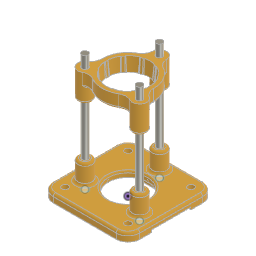
Drill_Guide_v7 (Autodesk Fusion 360 design; units mm, degrees)
Autodesk Fusion 360 part; units mm, degrees
sketch "Sketch1" plane through (0, 0, 0) normal (0, 0, 1) x (1, 0, 0) in component "Mount"
  circle A0 centre (0, 0) radius 32.75
  dimension "d45" = 65.5
  constraint coincident A0.centre origin
  measures "d45" diameter of A0
extrude "Extrude1" add sketch "Sketch1" along normal blind 17 makes body 1 in component "Mount"
sketch "Sketch3" plane through (0, 0, 0) normal (0, 0, -1) x (1, 0, 0) in component "Mount"
  circle A0 centre (0, 0) radius 32.75
  circle A1 centre (0, 0) radius 27.75
  line L0 (0, 0) -> (-27.75, 0) construction
  line L1 (-28.25, -2.5) -> (-28.25, -2.5)
  line L2 (-27.25, -1.5) -> (-27.25, 1.5)
  line L3 (-28.25, 2.5) -> (-28.25, 2.5)
  line L4 (-28.25, 2.5) -> (-28.25, -2.5)
  line L5 (-28.25, -2.5) -> (-27.25, 2.5) construction
  line L6 (-27.25, -2.5) -> (-28.25, 2.5) construction
  arc A2 (-27.25, 1.5) -> (-28.25, 2.5) centre (-28.25, 1.5) ccw
  arc A3 (-28.25, -2.5) -> (-27.25, -1.5) centre (-28.25, -1.5) ccw
  line L7 (-21.164, -17.2307) -> (-22.9274, -14.8036)
  arc A4 (-21.3853, -18.6275) -> (-21.164, -17.2307) centre (-21.9731, -17.8185) ccw
  arc A5 (-22.9274, -14.8036) -> (-24.3242, -14.5824) centre (-23.7364, -15.3914) ccw
  line L8 (-24.3242, -14.5824) -> (-21.3853, -18.6275)
  line L9 (-6.9941, -26.3798) -> (-9.8473, -25.4528)
  arc A6 (-6.3521, -27.6399) -> (-6.9941, -26.3798) centre (-7.3031, -27.3309) ccw
  arc A7 (-9.8473, -25.4528) -> (-11.1074, -26.0948) centre (-10.1563, -26.4038) ccw
  line L10 (-11.1074, -26.0948) -> (-6.3521, -27.6399)
  line L11 (9.8473, -25.4528) -> (6.9941, -26.3798)
  arc A8 (11.1074, -26.0948) -> (9.8473, -25.4528) centre (10.1563, -26.4038) ccw
  arc A9 (6.9941, -26.3798) -> (6.3521, -27.6399) centre (7.3031, -27.3309) ccw
  line L12 (6.3521, -27.6399) -> (11.1074, -26.0948)
  line L13 (22.9274, -14.8036) -> (21.164, -17.2307)
  arc A10 (24.3242, -14.5824) -> (22.9274, -14.8036) centre (23.7364, -15.3914) ccw
  arc A11 (21.164, -17.2307) -> (21.3853, -18.6275) centre (21.9731, -17.8185) ccw
  line L14 (21.3853, -18.6275) -> (24.3242, -14.5824)
  line L15 (27.25, 1.5) -> (27.25, -1.5)
  arc A12 (28.25, 2.5) -> (27.25, 1.5) centre (28.25, 1.5) ccw
  arc A13 (27.25, -1.5) -> (28.25, -2.5) centre (28.25, -1.5) ccw
  line L16 (28.25, -2.5) -> (28.25, 2.5)
  line L17 (21.164, 17.2307) -> (22.9274, 14.8036)
  arc A14 (21.3853, 18.6275) -> (21.164, 17.2307) centre (21.9731, 17.8185) ccw
  arc A15 (22.9274, 14.8036) -> (24.3242, 14.5824) centre (23.7364, 15.3914) ccw
  line L18 (24.3242, 14.5824) -> (21.3853, 18.6275)
  line L19 (6.9941, 26.3798) -> (9.8473, 25.4528)
  arc A16 (6.3521, 27.6399) -> (6.9941, 26.3798) centre (7.3031, 27.3309) ccw
  arc A17 (9.8473, 25.4528) -> (11.1074, 26.0948) centre (10.1563, 26.4038) ccw
  line L20 (11.1074, 26.0948) -> (6.3521, 27.6399)
  line L21 (-9.8473, 25.4528) -> (-6.9941, 26.3798)
  arc A18 (-11.1074, 26.0948) -> (-9.8473, 25.4528) centre (-10.1563, 26.4038) ccw
  arc A19 (-6.9941, 26.3798) -> (-6.3521, 27.6399) centre (-7.3031, 27.3309) ccw
  line L22 (-6.3521, 27.6399) -> (-11.1074, 26.0948)
  line L23 (-22.9274, 14.8036) -> (-21.164, 17.2307)
  arc A20 (-24.3242, 14.5824) -> (-22.9274, 14.8036) centre (-23.7364, 15.3914) ccw
  arc A21 (-21.164, 17.2307) -> (-21.3853, 18.6275) centre (-21.9731, 17.8185) ccw
  line L24 (-21.3853, 18.6275) -> (-24.3242, 14.5824)
  point P0 (-27.75, 0)
  dimension "d60" = 55.5
  dimension "d61" = 1
  dimension "d62" = 5
  dimension "d63" = 1
  dimension "d64" = 1
  dimension "d66" = 360
  constraint coincident A0.centre A1.centre
  constraint coincident A1 P0
  constraint horizontal L0
  constraint parallel L2 L4
  constraint coincident L5 P0
  constraint coincident L6 P0
  constraint coincident P0 L0.end
  constraint coincident L5.end L3
  constraint coincident L5.end L2
  constraint tangent L2 A2
  constraint coincident L6.start L1
  constraint coincident L6.start L2
  constraint tangent L2 A3
  measures "d60" diameter of A1
  measures "d61" distance of L5.end L3.start
  measures "d62" distance of L6.start L5.end
  measures "d63" radius of A2
  measures "d64" radius of A3
extrude "Extrude2" cut sketch "Sketch3" against normal up to surface (17 mm away) draft -5 contours A1 L2 A2 A3 L7 A4 A5 L9 A6 A7 L11 A8 A9 L13 A10 A11 L15 A12 A13 L17 A14 A15 L19 A16 A17 L21 A18 A19 L23 A20 A21 bodies 1 in component "Mount"
sketch "Sketch1 (2)" plane through (0, 0, 0) normal (0, 0, 1) x (1, 0, 0) in component "Base"
  circle A0 centre (-40, -40) radius 4
  line L0 (-55, 55) -> (55, -55) construction
  line L1 (55, 55) -> (-55, -55) construction
  arc A1 (-40, 55) -> (-55, 40) centre (-40, 40) ccw
  arc A2 (-55, -40) -> (-40, -55) centre (-40, -40) ccw
  line L2 (-55, -40) -> (-55, 40)
  circle A3 centre (-40, 40) radius 4
  line L3 (-40, 55) -> (40, 55)
  arc A4 (55, 40) -> (40, 55) centre (40, 40) ccw
  line L4 (55, 40) -> (55, -40)
  line L5 (40, -55) -> (-40, -55)
  circle A5 centre (40, -40) radius 4
  arc A6 (40, -55) -> (55, -40) centre (40, -40) ccw
  circle A7 centre (40, 40) radius 4
  circle A8 centre (0, 0) radius 25
  dimension "d69" = 110
  dimension "d70" = 110
  dimension "d71" = 15
  dimension "d72" = 15
  dimension "d73" = 15
  dimension "d74" = 15
  dimension "d75" = 8
  dimension "d76" = 8
  dimension "d77" = 8
  dimension "d78" = 8
  dimension "d79" = 50
  constraint horizontal L3
  constraint perpendicular L3 L4
  constraint parallel L3 L5
  constraint parallel L2 L4
  constraint coincident A8.centre L0
  constraint coincident A8.centre L1
  constraint coincident A8.centre origin
  constraint coincident L1.end L2
  constraint coincident L1.end L5
  constraint tangent A2 L2
  constraint tangent A2 L5
  constraint coincident L0.start L2
  constraint coincident L0.start L3
  constraint tangent A1 L2
  constraint tangent A1 L3
  constraint coincident L1.start L3
  constraint coincident L1.start L4
  constraint tangent L3 A4
  constraint tangent A4 L4
  constraint coincident L0.end L4
  constraint coincident L0.end L5
  constraint tangent L4 A6
  constraint tangent L5 A6
  constraint concentric A0 A2
  constraint concentric A5 A6
  constraint concentric A4 A7
  constraint concentric A1 A3
  measures "d69" distance of L0.end L1.end
  measures "d70" distance of L0.end L1.start
  measures "d71" radius of A2
  measures "d72" radius of A1
  measures "d73" radius of A4
  measures "d74" radius of A6
  measures "d75" diameter of A0
  measures "d76" diameter of A5
  measures "d77" diameter of A7
  measures "d78" diameter of A3
  measures "d79" diameter of A8
extrude "Extrude1'" add sketch "Sketch1 (2)" along normal blind 10 separate body makes body 2 in component "Base"
sketch "Sketch2" plane through (55, 0, 0) normal (1, 0, 0) x (0, 1, 0) in component "Base"
  line L0 (-40, 0) -> (40, 0)
  line L1 (40, 0) -> (40, 10)
  line L2 (40, 10) -> (-40, 10)
  line L3 (-40, 10) -> (-40, 0)
  line L4 (25, 0) -> (-25, 0)
  line L5 (25, 3) -> (25, 0)
  line L6 (-40, 0) -> (40, 0)
  line L7 (40, 0) -> (40, 10)
  line L8 (40, 10) -> (-40, 10)
  line L9 (-40, 10) -> (-40, 0)
  line L10 (-25, 0) -> (-25, 3)
  line L11 (-25, 3) -> (25, 3)
  dimension "d82" = 50
  dimension "d83" = 3
  constraint horizontal L11
  constraint vertical L5
  constraint horizontal L4
  constraint vertical L10
  constraint midpoint origin L4
  measures "d82" distance of L10.end L5.start
  measures "d83" distance of L10.end L4.end
extrude "Extrude2'" cut sketch "Sketch2" against normal up to surface (110 mm away) contours L0 L4 L5 L6 L10 L11 bodies 2 in component "Base"
sketch "Sketch3 (2)" plane through (0, 0, 10) normal (0, 0, 1) x (-1, 0, 0) in component "Base"
  circle A0 centre (-40, -40) radius 4
  circle A1 centre (0, 0) radius 25
  circle A2 centre (40, 40) radius 4
  circle A3 centre (40, -40) radius 4
  circle A4 centre (-40, 40) radius 4
  arc A5 (55, 40) -> (40, 55) centre (40, 40) ccw
  line L0 (40, 55) -> (-40, 55)
  arc A6 (-40, 55) -> (-55, 40) centre (-40, 40) ccw
  line L1 (-55, 40) -> (-55, -40)
  arc A7 (-55, -40) -> (-40, -55) centre (-40, -40) ccw
  line L2 (-40, -55) -> (40, -55)
  arc A8 (40, -55) -> (55, -40) centre (40, -40) ccw
  line L3 (55, -40) -> (55, 40)
  circle A9 centre (0, 0) radius 25
  circle A10 centre (40, 40) radius 4
  circle A11 centre (-40, 40) radius 4
  circle A12 centre (-40, -40) radius 4
  arc A13 (40, -55) -> (55, -40) centre (40, -40) ccw
  circle A14 centre (0, -40) radius 9
  circle A15 centre (-34.641, 20) radius 9
  circle A16 centre (34.641, 20) radius 9
  line L4 (-40, -55) -> (40, -55)
  circle A17 centre (40, -40) radius 4
  line L5 (40, 55) -> (-40, 55)
  line L6 (55, -40) -> (55, 40)
  arc A18 (55, 40) -> (40, 55) centre (40, 40) ccw
  arc A19 (-40, 55) -> (-55, 40) centre (-40, 40) ccw
  line L7 (-55, 40) -> (-55, -40)
  arc A20 (-55, -40) -> (-40, -55) centre (-40, -40) ccw
  dimension "d87" = 360
  dimension "d88" = 40
  dimension "d89" = 55
  measures "d88" distance of A14.centre A1.centre
  measures "d89" distance of A14.centre L6
extrude "Extrude3" add sketch "Sketch3 (2)" along normal blind 25 contours A14 | A15 | A16 bodies 2 in component "Base"
sketch "Sketch4" plane through (0, 0, 35) normal (0, 0, 1) x (-1, 0, 0) in component "Base"
  circle A0 centre (0, -40) radius 9
  circle A1 centre (34.641, 20) radius 4
  circle A2 centre (-34.641, 20) radius 4
  circle A3 centre (0, -40) radius 4
  circle A4 centre (0, -40) radius 9
  dimension "d93" = 360
  dimension "d94" = 8
  constraint concentric A3 A4
  measures "d94" diameter of A3
extrude "Extrude4" cut sketch "Sketch4" against normal up to surface (35 mm away) contours A1 | A2 | A3 bodies 2 in component "Base"
ref_plane "WorkPlane1" through (0, 0, 3) normal (0, 0, 1) x (1, 0, 0) in component "Base"
sketch "Sketch5" plane through (0, 0, 3) normal (0, 0, 1) x (1, 0, 0) in component "Base"
  circle A0 centre (25, 0) radius 0.5
  circle A1 centre (0, -25) radius 0.5
  circle A2 centre (0, 25) radius 0.5
  circle A3 centre (-25, 0) radius 0.5
  dimension "d99" = 360
  dimension "d100" = 1
  measures "d100" diameter of A2
extrude "Extrude5" add sketch "Sketch5" along normal blind 3 bodies 2 in component "Base"
fillet "Fillet1" radius 3 11 edges at (55, 0, 10) (50.6066, 50.6066, 10) (0, 55, 10) (-50.6066, 50.6066, 10) (-55, 0, 10) (-50.6066, -50.6066, 10) (0, -55, 10) (50.6066, -50.6066, 10) (43.032, -16.7455, 35) (8.3909, 43.2545, 35) (-26.2501, -16.7455, 35) on bodies 2 in component "Base"
fillet "Fillet3" radius 2 1 edges at (-23.3082, 9.0404, 10) on bodies 2 in component "Base"
fillet "Fillet4" radius 3 3 edges at (-26.2501, -23.2545, 10) (8.3909, 36.7455, 10) (43.032, -23.2545, 10) on bodies 2 in component "Base"
sketch "Sketch4 (2)" plane through (0, 0, 0) normal (0, 0, -1) x (1, 0, 0) in component "Mount"
  arc A0 (23.7265, -14.3915) -> (27.6543, -2.3032) centre (0, 0) ccw
  arc A1 (23.7265, -14.3915) -> (22.9274, -14.8036) centre (23.7364, -15.3914) ccw
  line L0 (22.9274, -14.8036) -> (21.164, -17.2307)
  arc A2 (21.164, -17.2307) -> (21.019, -18.1181) centre (21.9731, -17.8185) ccw
  arc A3 (10.7361, -25.589) -> (21.019, -18.1181) centre (0, 0) ccw
  arc A4 (10.7361, -25.589) -> (9.8473, -25.4528) centre (10.1563, -26.4038) ccw
  line L1 (9.8473, -25.4528) -> (6.9941, -26.3798)
  arc A5 (6.9941, -26.3798) -> (6.3552, -27.0125) centre (7.3031, -27.3309) ccw
  arc A6 (-6.3552, -27.0125) -> (6.3552, -27.0125) centre (0, 0) ccw
  arc A7 (-6.3552, -27.0125) -> (-6.9941, -26.3798) centre (-7.3031, -27.3309) ccw
  line L2 (-6.9941, -26.3798) -> (-9.8473, -25.4528)
  arc A8 (-9.8473, -25.4528) -> (-10.7361, -25.589) centre (-10.1563, -26.4038) ccw
  arc A9 (-21.019, -18.1181) -> (-10.7361, -25.589) centre (0, 0) ccw
  arc A10 (-21.019, -18.1181) -> (-21.164, -17.2307) centre (-21.9731, -17.8185) ccw
  line L3 (-21.164, -17.2307) -> (-22.9274, -14.8036)
  arc A11 (-22.9274, -14.8036) -> (-23.7265, -14.3915) centre (-23.7364, -15.3914) ccw
  arc A12 (-27.6543, -2.3032) -> (-23.7265, -14.3915) centre (0, 0) ccw
  arc A13 (-27.6543, -2.3032) -> (-27.25, -1.5) centre (-28.25, -1.5) ccw
  line L4 (-27.25, -1.5) -> (-27.25, 1.5)
  arc A14 (-27.25, 1.5) -> (-27.6543, 2.3032) centre (-28.25, 1.5) ccw
  arc A15 (-23.7265, 14.3915) -> (-27.6543, 2.3032) centre (0, 0) ccw
  arc A16 (-23.7265, 14.3915) -> (-22.9274, 14.8036) centre (-23.7364, 15.3914) ccw
  line L5 (-22.9274, 14.8036) -> (-21.164, 17.2307)
  arc A17 (-21.164, 17.2307) -> (-21.019, 18.1181) centre (-21.9731, 17.8185) ccw
  arc A18 (-10.7361, 25.589) -> (-21.019, 18.1181) centre (0, 0) ccw
  arc A19 (-10.7361, 25.589) -> (-9.8473, 25.4528) centre (-10.1563, 26.4038) ccw
  line L6 (-9.8473, 25.4528) -> (-6.9941, 26.3798)
  arc A20 (-6.9941, 26.3798) -> (-6.3552, 27.0125) centre (-7.3031, 27.3309) ccw
  arc A21 (6.3552, 27.0125) -> (-6.3552, 27.0125) centre (0, 0) ccw
  arc A22 (6.3552, 27.0125) -> (6.9941, 26.3798) centre (7.3031, 27.3309) ccw
  line L7 (6.9941, 26.3798) -> (9.8473, 25.4528)
  arc A23 (9.8473, 25.4528) -> (10.7361, 25.589) centre (10.1563, 26.4038) ccw
  arc A24 (21.019, 18.1181) -> (10.7361, 25.589) centre (0, 0) ccw
  arc A25 (21.019, 18.1181) -> (21.164, 17.2307) centre (21.9731, 17.8185) ccw
  line L8 (21.164, 17.2307) -> (22.9274, 14.8036)
  arc A26 (22.9274, 14.8036) -> (23.7265, 14.3915) centre (23.7364, 15.3914) ccw
  arc A27 (27.6543, 2.3032) -> (23.7265, 14.3915) centre (0, 0) ccw
  arc A28 (27.6543, 2.3032) -> (27.25, 1.5) centre (28.25, 1.5) ccw
  line L9 (27.25, 1.5) -> (27.25, -1.5)
  arc A29 (27.25, -1.5) -> (27.6543, -2.3032) centre (28.25, -1.5) ccw
  circle A30 centre (0, 0) radius 32.75
  circle A31 centre (0, -40) radius 9
  circle A32 centre (34.641, 20) radius 4.05
  circle A33 centre (-34.641, 20) radius 4.05
  circle A34 centre (0, -40) radius 9
  circle A35 centre (0, -40) radius 4.05
  circle A36 centre (34.641, 20) radius 9
  circle A37 centre (-34.641, 20) radius 9
  dimension "d112" = 360
  dimension "d113" = 8.1
  dimension "d114" = 18
  dimension "d115" = 18
  constraint concentric A34 A35
  constraint concentric A32 A36
  constraint concentric A33 A37
  measures "d113" diameter of A35
  measures "d114" diameter of A36
  measures "d115" diameter of A37
extrude "Extrude3'" add sketch "Sketch4 (2)" against normal blind 35 contours A30 A36 | A30 A36 | A30 A31 A34 | A30 A31 A34 | A30 A37 | A30 A37 bodies 1 in component "Mount"
fillet "Fillet1'" radius 14 6 edges at (-25.6484, -20.3647, 8.5) (4.8122, 32.3945, 8.5) (-4.8122, 32.3945, 8.5) (-30.4606, -12.0298, 8.5) (25.6484, -20.3647, 8.5) (30.4606, -12.0298, 8.5) on bodies 1 in component "Mount"
fillet "Fillet2" radius 3 12 edges at (-43.032, -23.2545, 35) (-8.3909, 36.7455, 35) (26.2501, -23.2545, 35) (-11.0081, 33.4645, 17) (-28.3623, 16.375, 17) (-34.4851, -7.1989, 17) (-23.477, -26.2655, 17) (0, -32.75, 17) (23.477, -26.2655, 17) (34.4851, -7.1989, 17) (28.3623, 16.375, 17) (11.0081, 33.4645, 17) on bodies 1 in component "Mount"
move_body "Move6" bodies 1 to x (-1, 0, 0) y (0, -1, 0) z (0, 0, 1) at (-69.282, -40, 0) in component "Mount"
sketch "Sketch1 (3)" plane through (0, 0, 0) normal (0, 0, 1) x (1, 0, 0) in component "rods"
  circle A0 centre (0, 40) radius 4
  circle A1 centre (-34.641, -20) radius 4
  circle A2 centre (34.641, -20) radius 4
  dimension "d136" = 8
  dimension "d141" = 360
  measures "d136" diameter of A0
extrude "Extrude2''" add sketch "Sketch1 (3)" along normal blind 150 separate body makes body 3 at (3.995, 39.8006, 100) makes body 4 at (-30.646, -20.1994, 100) makes body 5 at (38.636, -20.1994, 100) in component "rods"
component "Base" placed x (1, 0, 0) y (0, 1, 0) z (0, 0, 1) at (0, 0, 0)
component "Mount" placed x (1, 0, 0) y (0, -1, 0) z (0, 0, -1) at (69.282, -40, 135)
component "rods" placed x (1, 0, 0) y (0, 1, 0) z (0, 0, 1) at (0, 0, 0)
